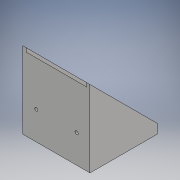
# Autodesk Inventor part: A0006
Saved by Autodesk Inventor 2017 (Build 210142000, 142)
## iProperties
Part Number: A0006
Material: 一般
Document SubType Name: Modeling
Designer: lygfy
Density: 1 g/cm^3
Appearance: 預設
Author: lygfy
Autodesk Inventor part; units mm, degrees
ref_plane "YZ Plane" through (0, 0, 0) normal (1, 0, 0) x (0, 1, 0)
ref_plane "XZ Plane" through (0, 0, 0) normal (0, 1, 0) x (-1, 0, 0)
ref_plane "XY Plane" through (0, 0, 0) normal (0, 0, 1) x (1, 0, 0)
sketch "草圖1" plane through (0, 0, 0) normal (1, 0, 0) x (0, 1, 0)
  line L0 (38.8909, -31.8198) -> (35.3553, -35.3553)
  line L1 (35.3553, -35.3553) -> (-35.3553, 35.3553)
  line L2 (-35.3553, 35.3553) -> (-31.8198, 38.8909)
  line L3 (-31.8198, 38.8909) -> (38.8909, -31.8198)
  line L4 (-50.2046, 0) -> (53.7401, 0) construction
  point P0 (0, 0)
  dimension "d0" = 45
  dimension "d1" = 5
  dimension "d2" = 100
  constraints: 8 end point, 2 parallel, 1 midpoint, 1 perpendicular
  measures "d0" angle of L4 L1
  measures "d1" distance of L0.start L0.end
  measures "d2" distance of L0.end L1.end
extrude "擠出1" add sketch "草圖1" along normal mid plane 50
sketch "草圖2" plane through (25, 38.8909, -31.8198) normal (0, 0.7071068, -0.7071068) x (-1, 0, 0)
  line L0 (50, 0) -> (0, 0) projected
  line L1 (47.5, 0) -> (2.5, 0)
  line L2 (2.5, 0) -> (2.5, -2)
  line L3 (2.5, -2) -> (47.5, -2)
  line L4 (47.5, -2) -> (47.5, 0)
  line L5 (0, -5) -> (50, -5) projected
  point P0 (25, -5)
  point P1 (25, -5)
  point P2 (25, -2)
  dimension "d5" = 45
  dimension "d6" = 2
  constraints: 8 end point, 2 midpoint, 2 parallel, 1 horizontal, 1 perpendicular, 1 point on line, 1 vertical alignment
  measures "d5" distance of L2.end L3.end
  measures "d6" distance of L3.end L1.start
extrude "擠出2" cut sketch "草圖2" against normal through all
sketch "草圖3" plane through (0, 0, 0) normal (1, 0, 0) x (0, 1, 0)
  line L0 (25, 68.2254) -> (-25, 68.2254)
  line L1 (-25, 68.2254) -> (-25, -53.4772)
  line L2 (-25, -53.4772) -> (25, -53.4772)
  line L3 (25, -53.4772) -> (25, 68.2254)
  point P0 (0, 0)
  point P1 (0, -53.4772)
  dimension "d9" = 50
  constraints: 8 end point, 2 parallel, 1 horizontal, 1 midpoint, 1 perpendicular, 1 vertical alignment
  measures "d9" distance of L0.start L0.end
extrude "擠出3" cut sketch "草圖3" along normal through all both and the other way through all keep common part
sketch "草圖4" plane through (0, 0, 0) normal (1, 0, 0) x (0, 1, 0)
  line L0 (-25, 25) -> (25, -25) projected
  line L1 (25, -25) -> (-25, -25)
  line L2 (-25, -25) -> (-25, 25)
  point P0 (0, 0)
  constraints: 4 end point, 2 vertical, 1 coincident, 1 horizontal, 1 point on line, 2 other
extrude "擠出4" add sketch "草圖4" against normal up to surface (50 mm away) from surface at 25
sketch "草圖5" plane through (-22.5, -25, 29.2426) normal (0, -1, 0) x (1, 0, 0)
  line L0 (37.5, -33.2426) -> (7.5, -33.2426)
  line L1 (-2.5, -54.2426) -> (47.5, -54.2426) projected
  point P0 (22.5, -29.2426)
  point P1 (22.5, -33.2426)
  dimension "d15" = 30
  dimension "d24" = 21
  constraints: 2 end point, 1 horizontal, 1 midpoint, 1 vertical alignment
  measures "d15" distance of L0.start L0.end
  measures "d24" distance between parallel lines of L0 L1
hole "孔1" at (15, -25, -4) at (-15, -25, -4) direction (0, 1, 0) diameter 2.459 depth 8.8 tip angle 118 thread size "M3x0.5" class "6H" standard "ISO Metric profile"
